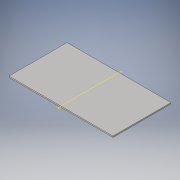
# Autodesk Inventor part: Back Plate
Saved by Autodesk Inventor 2016 SP2 (Build 200236200, 236)
## iProperties
Created: 2018-01-31
Part Number: Back Plate
Material: Generic
Document SubType Name: Modeling
Designer: CAD
Density: 1 g/cm^3
Appearance: Default
Author: CAD
Autodesk Inventor part; units mm, degrees
ref_plane "XZ Plane" through (0, 0, 0) normal (0, 1, 0) x (-1, 0, 0)
ref_plane "XY Plane" through (0, 0, 0) normal (0, 0, 1) x (1, 0, 0)
sketch "Sketch1" plane through (0, 0, 0) normal (0, 1, 0) x (-1, 0, 0)
  line L0 (136.525, 76.2) -> (-136.525, 76.2)
  line L1 (-136.525, 76.2) -> (-136.525, -76.2)
  line L2 (-136.525, -76.2) -> (136.525, -76.2)
  line L3 (136.525, -76.2) -> (136.525, 76.2)
  point P0 (0, 0)
  dimension "d0" = 152.4
  dimension "d1" = 273.05
  dimension "d2" = 136.525
  dimension "d3" = 76.2
  constraints: 8 end point, 2 parallel, 1 horizontal, 1 perpendicular
  measures "d0" distance of L2.end L0.start
  measures "d1" distance of L0.start L0.end
  measures "d2" distance from line of L3 point (0, 0)
  measures "d3" distance from line of L0 point (0, 0)
extrude "Extrusion1" add sketch "Sketch1" along normal blind 3.175
body "Solid1"
